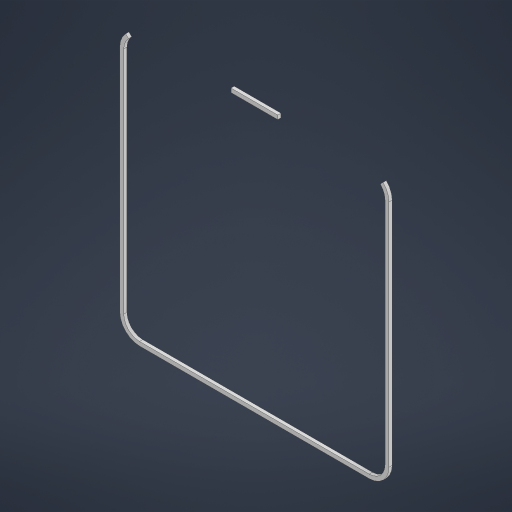
# Autodesk Inventor part: sumec_box-seal
Saved by Autodesk Inventor 2024 (Build 280153000, 153)
## iProperties
Created: 2024-03-06
Part Number: sumec_box-seal
Material: Všeobecné
Document SubType Name: Modeling
Designer: Simak
Density: 1 g/cm^3
Appearance: Výchozí
Author: Simak
Autodesk Inventor part; units mm, degrees
ref_plane "YZ Plane" through (0, 0, 0) normal (1, 0, 0) x (0, 1, 0)
ref_plane "XZ Plane" through (0, 0, 0) normal (0, 1, 0) x (-1, 0, 0)
ref_plane "XY Plane" through (0, 0, 0) normal (0, 0, 1) x (1, 0, 0)
sketch "Náčrt1" plane through (0, 0, 0) normal (0, 0, 1) x (1, 0, 0)
  line L0 (-46.5, 54.5) -> (46.5, 54.5)
  line L1 (54.5, 46.5) -> (54.5, -46.5)
  line L2 (46.5, -54.5) -> (-46.5, -54.5)
  line L3 (-54.5, -46.5) -> (-54.5, 46.5)
  line L4 (-54.5, 54.5) -> (0, 0) construction
  line L5 (0, 0) -> (54.5, 54.5) construction
  line L6 (54.5, -54.5) -> (0, 0) construction
  arc A0 (-46.5, 54.5) -> (-54.5, 46.5) centre (-46.5, 46.5) ccw
  arc A1 (-54.5, -46.5) -> (-46.5, -54.5) centre (-46.5, -46.5) ccw
  arc A2 (46.5, -54.5) -> (54.5, -46.5) centre (46.5, -46.5) ccw
  arc A3 (54.5, 46.5) -> (46.5, 54.5) centre (46.5, 46.5) ccw
  line L7 (46.5, 53.7) -> (-46.5, 53.7) construction
  arc A4 (-46.5, 53.7) -> (-53.7, 46.5) centre (-46.5, 46.5) ccw construction
  line L8 (-53.7, 46.5) -> (-53.7, -46.5) construction
  arc A5 (-53.7, -46.5) -> (-46.5, -53.7) centre (-46.5, -46.5) ccw construction
  line L9 (-46.5, -53.7) -> (46.5, -53.7) construction
  arc A6 (46.5, -53.7) -> (53.7, -46.5) centre (46.5, -46.5) ccw construction
  line L10 (53.7, -46.5) -> (53.7, 46.5) construction
  arc A7 (53.7, 46.5) -> (46.5, 53.7) centre (46.5, 46.5) ccw construction
  line L11 (46.5, -52.9) -> (-46.5, -52.9)
  arc A8 (-52.9, -46.5) -> (-46.5, -52.9) centre (-46.5, -46.5) ccw
  line L12 (-52.9, -46.5) -> (-52.9, 46.5)
  arc A9 (-46.5, 52.9) -> (-52.9, 46.5) centre (-46.5, 46.5) ccw
  line L13 (-46.5, 52.9) -> (46.5, 52.9)
  arc A10 (52.9, 46.5) -> (46.5, 52.9) centre (46.5, 46.5) ccw
  line L14 (52.9, 46.5) -> (52.9, -46.5)
  arc A11 (46.5, -52.9) -> (52.9, -46.5) centre (46.5, -46.5) ccw
  line L15 (-46.5, 55.7) -> (46.5, 55.7) construction
  arc A12 (55.7, 46.5) -> (46.5, 55.7) centre (46.5, 46.5) ccw construction
  line L16 (55.7, 46.5) -> (55.7, -46.5) construction
  arc A13 (46.5, -55.7) -> (55.7, -46.5) centre (46.5, -46.5) ccw construction
  line L17 (46.5, -55.7) -> (-46.5, -55.7) construction
  arc A14 (-55.7, -46.5) -> (-46.5, -55.7) centre (-46.5, -46.5) ccw construction
  line L18 (-55.7, -46.5) -> (-55.7, 46.5) construction
  arc A15 (-46.5, 55.7) -> (-55.7, 46.5) centre (-46.5, 46.5) ccw construction
  line L19 (-54.5, 53) -> (54.5, 53) construction
  line L20 (46.5, 46.5) -> (52.1134, 52.2)
  line L21 (-46.5, 46.5) -> (-52.1134, 52.2)
  line L22 (9.4667, 52.9) -> (9.4667, 55.7)
  line L23 (-9.4667, 52.9) -> (-9.4667, 54.5)
  point P0 (50.9907, 51.06)
  point P1 (-50.9907, 51.06)
  point P2 (9.4667, 54.5)
  dimension "d0" = 109
  dimension "d1" = 109
  dimension "d2" = 8
  dimension "d3" = 0.8
  dimension "d4" = 0.8
  dimension "d5" = 2
  dimension "d6" = 2.7
  dimension "d7" = 0.8
  dimension "d8" = 0.8
  dimension "d10" = 37.0333
  dimension "d13" = 37.0333
  constraints: 48 end point, 34 point on circle, 16 centre point, 10 point on line, 9 parallel, 8 tangent, 6 perpendicular, 3 equal radius, 2 equal length, 2 vertical alignment, 1 horizontal, 21 other
  measures "d0" distance of L5.end L6.start
  measures "d1" distance of L4.start L5.end
  measures "d2" radius of A0
  measures "d3" distance between parallel lines of L0 L7
  measures "d4" distance between parallel lines of L9 L11
  measures "d5" distance between parallel lines of L7 L15
  measures "d6" distance between parallel lines of L15 L19
  measures "d7" distance from line of L19 L20.end
  measures "d8" distance from line of L19 L21.end
  measures "d10" distance from line of L13.end L22
  measures "d13" distance from line of L23 L0.start
extrude "Vysunutí1" add sketch "Náčrt1" along normal blind 1.3 contours L0 L22 L13 L23 | L21 A9 L12 A8 L11 A11 L14 A10 L20 A3 L1 A2 L2 A1 L3 A0
equation "\"d1\" = d0"
equation "\"d4\" = d3"
equation "\"d8\" = d7"
equation "\"d13\" = d10"
